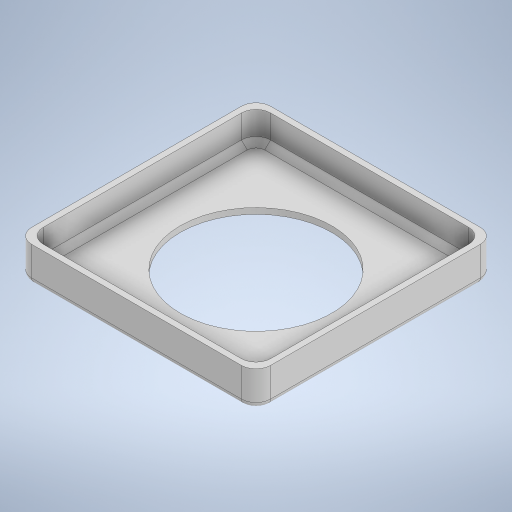
# Autodesk Inventor part: controler_03
Saved by Autodesk Inventor 2023 (Build 270158000, 158)
## iProperties
Created: 2023-10-10
Part Number: controler_03
Material: Generic
Document SubType Name: Modeling
Designer: Michal
Density: 1 g/cm^3
Appearance: Default
Author: Michal
Autodesk Inventor part; units mm, degrees
ref_plane "YZ Plane" through (0, 0, 0) normal (1, 0, 0) x (0, 1, 0)
ref_plane "XZ Plane" through (0, 0, 0) normal (0, 1, 0) x (-1, 0, 0)
ref_plane "XY Plane" through (0, 0, 0) normal (0, 0, 1) x (1, 0, 0)
sketch "Sketch1" plane through (0, 0, 0) normal (0, 1, 0) x (-1, 0, 0)
  line L0 (28.931, 30.3524) -> (-43.069, 30.3524)
  line L1 (-48.069, 25.3524) -> (-48.069, -51.6476)
  line L2 (-43.069, -51.6476) -> (33.931, -51.6476)
  line L3 (33.931, -46.6476) -> (33.931, 30.3524)
  arc A0 (-48.069, -46.6476) -> (-43.069, -51.6476) centre (-43.069, -46.6476) ccw
  line L4 (-46.069, 28.3524) -> (26.931, 28.3524)
  line L5 (31.931, 23.3524) -> (31.931, -44.6476)
  line L6 (31.931, -49.6476) -> (-46.069, -49.6476)
  line L7 (-46.069, -44.6476) -> (-46.069, 23.3524)
  arc A1 (-38.6778, 27.7435) -> (-45.4601, 20.9612) centre (-41.069, 23.3524) ccw
  arc A2 (24.5399, -49.0388) -> (31.3222, -42.2565) centre (26.931, -44.6476) ccw
  arc A3 (31.3222, 20.9612) -> (24.5399, 27.7435) centre (26.931, 23.3524) ccw
  arc A4 (-45.4601, -42.2565) -> (-38.6778, -49.0388) centre (-41.069, -44.6476) ccw
  arc A5 (33.931, 25.3524) -> (28.931, 30.3524) centre (28.931, 25.3524) ccw
  arc A6 (-46.069, 21.3524) -> (-45.4601, 20.9612) centre (-43.069, 25.3524) ccw
  arc A7 (-43.069, 30.3524) -> (-48.069, 25.3524) centre (-43.069, 25.3524) ccw
  arc A8 (28.931, -51.6476) -> (33.931, -46.6476) centre (28.931, -46.6476) ccw
  point P0 (0, 0)
  point P1 (-41.069, -49.6476)
  point P2 (26.931, -49.6476)
  point P3 (-41.069, 28.3524)
  dimension "d0" = 82
  dimension "d1" = 82
  dimension "d3" = 10
  dimension "d7" = 78
  dimension "d8" = 78
  dimension "d9" = 2
  dimension "d10" = 2
  dimension "d11" = 10
  dimension "d12" = 10
  dimension "d13" = 10
  dimension "d14" = 10
  constraints: 23 point on circle, 16 end point, 16 tangent, 9 centre point, 4 parallel, 4 point on line, 2 horizontal, 2 perpendicular
  measures "d0" distance of L2.end L3.end
  measures "d1" distance of L1.end L2.end
  measures "d3" diameter of A0
  measures "d7" distance of L6.start L6.end
  measures "d8" distance of L6.end L4.start
  measures "d9" distance between parallel lines of L2 L6
  measures "d10" distance between parallel lines of L1 L7
  measures "d11" diameter of A1
  measures "d12" diameter of A2
  measures "d13" diameter of A3
  measures "d14" diameter of A4
extrude "Extrusion1" add sketch "Sketch1" along normal blind 2 contours L4 A3 L5 A2 L6 A4 L7 A6 A1
extrude "Extrusion2" add sketch "Sketch1" along normal blind 15
sketch "Sketch2" plane through (0, 0, 0) normal (0, -1, 0) x (1, 0, 0)
  line L0 (48.069, 25.3524) -> (48.069, -46.6476) projected
  arc A0 (48.069, 25.3524) -> (43.069, 30.3524) centre (43.069, 25.3524) ccw projected
  line L1 (-28.931, 30.3524) -> (43.069, 30.3524) projected
  arc A1 (-28.931, 30.3524) -> (-33.931, 25.3524) centre (-28.931, 25.3524) ccw projected
  line L2 (-33.931, -46.6476) -> (-33.931, 25.3524) projected
  arc A2 (-33.931, -46.6476) -> (-28.931, -51.6476) centre (-28.931, -46.6476) ccw projected
  line L3 (43.069, -51.6476) -> (-28.931, -51.6476) projected
  arc A3 (43.069, -51.6476) -> (48.069, -46.6476) centre (43.069, -46.6476) ccw projected
  arc A4 (45.4601, 20.9612) -> (46.069, 21.3524) centre (43.069, 25.3524) ccw projected
  arc A5 (45.4601, 20.9612) -> (46.069, 23.3524) centre (41.069, 23.3524) ccw projected
  line L4 (46.069, 21.3524) -> (46.069, 23.3524) projected
  circle A6 centre (7.069, -10.6476) radius 26
  point P0 (0, 0)
  dimension "d19" = 52
  constraints: 1 centre point, 1 coincident
  measures "d19" diameter of A6
extrude "Extrusion3" cut sketch "Sketch2" along normal mid plane 15 contours A6
sketch "Sketch3" plane through (0, 15, 0) normal (0, 1, 0) x (1, 0, 0)
  line L0 (48.069, -25.3524) -> (48.069, 46.6476) projected
  arc A0 (48.069, 46.6476) -> (43.069, 51.6476) centre (43.069, 46.6476) ccw projected
  line L1 (43.069, 51.6476) -> (-28.931, 51.6476) projected
  arc A1 (-28.931, 51.6476) -> (-33.931, 46.6476) centre (-28.931, 46.6476) ccw projected
  line L2 (-33.931, 46.6476) -> (-33.931, -25.3524) projected
  arc A2 (-33.931, -25.3524) -> (-28.931, -30.3524) centre (-28.931, -25.3524) ccw projected
  line L3 (-28.931, -30.3524) -> (43.069, -30.3524) projected
  arc A3 (43.069, -30.3524) -> (48.069, -25.3524) centre (43.069, -25.3524) ccw projected
  arc A4 (46.069, 44.6476) -> (41.069, 49.6476) centre (41.069, 44.6476) ccw projected
  line L4 (46.069, 44.6476) -> (46.069, -23.3524) projected
  arc A5 (41.069, -28.3524) -> (46.069, -23.3524) centre (41.069, -23.3524) ccw projected
  line L5 (41.069, -28.3524) -> (-26.931, -28.3524) projected
  arc A6 (-31.931, -23.3524) -> (-26.931, -28.3524) centre (-26.931, -23.3524) ccw projected
  line L6 (-31.931, -23.3524) -> (-31.931, 44.6476) projected
  arc A7 (-26.931, 49.6476) -> (-31.931, 44.6476) centre (-26.931, 44.6476) ccw projected
  line L7 (-26.931, 49.6476) -> (41.069, 49.6476) projected
  point P0 (0, 0)
extrude "Extrusion4" cut sketch "Sketch3" against normal blind 3
fillet "Fillet1" radius 2 8 edges at (7.069, 0, -51.6476) (-32.4666, 0, -50.1832) (-33.931, 0, -10.6476) (-32.4666, 0, 28.8879) (7.069, 0, 30.3524) (46.6045, 0, 28.8879) (48.069, 0, -10.6476) (46.6045, 0, -50.1832)
sketch "Sketch4" plane through (0, 0, 0) normal (0, -1, 0) x (1, 0, 0)
  line L0 (46.069, 21.3524) -> (46.069, -46.6476) projected
  arc A0 (45.4601, 20.9612) -> (46.069, 21.3524) centre (43.069, 25.3524) ccw projected
  arc A1 (45.4601, 20.9612) -> (46.069, 23.3524) centre (41.069, 23.3524) ccw projected
  line L1 (46.069, 25.3524) -> (46.069, 23.3524) projected
  arc A2 (46.069, 25.3524) -> (43.069, 28.3524) centre (43.069, 25.3524) ccw projected
  line L2 (-28.931, 28.3524) -> (43.069, 28.3524) projected
  arc A3 (-28.931, 28.3524) -> (-31.931, 25.3524) centre (-28.931, 25.3524) ccw projected
  line L3 (-31.931, -46.6476) -> (-31.931, 25.3524) projected
  arc A4 (-31.931, -46.6476) -> (-28.931, -49.6476) centre (-28.931, -46.6476) ccw projected
  line L4 (43.069, -49.6476) -> (-28.931, -49.6476) projected
  arc A5 (43.069, -49.6476) -> (46.069, -46.6476) centre (43.069, -46.6476) ccw projected
  circle A6 centre (7.069, -10.6476) radius 26 projected
  line L5 (46.069, 23.3524) -> (46.069, -44.6476) projected
  line L6 (46.069, 21.3524) -> (46.069, 23.3524)
  point P0 (0, 0)
  constraints: 2 end point, 1 collinear, 1 tangent
extrude "Extrusion5" add sketch "Sketch4" against normal blind 2 contours A0 A1 L5
chamfer "Chamfer1" distance 2 angle 45 8 edges at (46.069, 2, -10.6476) (44.6045, 2, 26.8879) (7.069, 2, 28.3524) (-30.4666, 2, 26.8879) (-31.931, 2, -10.6476) (-30.4666, 2, -48.1832) (7.069, 2, -49.6476) (44.6045, 2, -48.1832)
body "Solid1"
